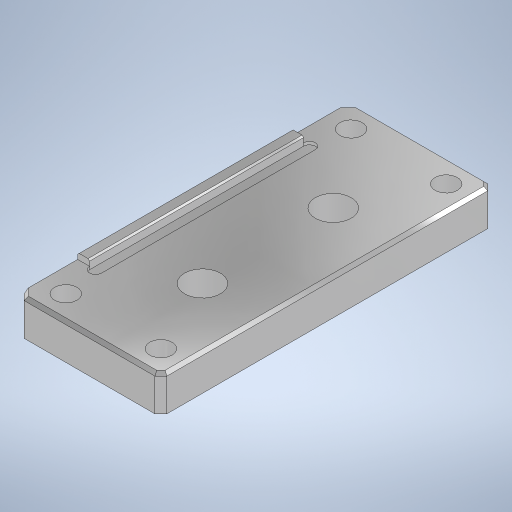
# Autodesk Inventor part: Base - Stationary
Saved by Autodesk Inventor 2023.2 (Build 272271000, 271)
## iProperties
Created: 2024-03-01
Part Number: Base - Stationary
Material: Aluminum 6061
Document SubType Name: Modeling
Designer: Nathan Cai
Density: 2.7 g/cm^3
Appearance: Aluminum - Flat
Author: Nathan Cai
Autodesk Inventor part; units mm, degrees
ref_plane "YZ Plane" through (0, 0, 0) normal (1, 0, 0) x (0, 1, 0)
ref_plane "XZ Plane" through (0, 0, 0) normal (0, 1, 0) x (-1, 0, 0)
ref_plane "XY Plane" through (0, 0, 0) normal (0, 0, 1) x (1, 0, 0)
sketch "Sketch1" plane through (0, 0, 0) normal (0, 1, 0) x (-1, 0, 0)
  line L0 (19.05, 44.45) -> (-19.05, 44.45)
  line L1 (-19.05, 44.45) -> (-19.05, -44.45)
  line L2 (-19.05, -44.45) -> (19.05, -44.45)
  line L3 (19.05, -44.45) -> (19.05, 44.45)
  line L4 (19.05, 44.45) -> (-19.05, -44.45) construction
  line L5 (-19.05, 44.45) -> (19.05, -44.45) construction
  line L6 (19.05, 0) -> (-19.05, 0) construction
  line L7 (0, 44.45) -> (0, -44.45) construction
  line L8 (19.05, 38.1) -> (-19.05, 38.1) construction
  circle A0 centre (-12.7, 38.1) radius 3
  circle A1 centre (12.7, 38.1) radius 3
  circle A2 centre (-12.7, -38.1) radius 3
  circle A3 centre (12.7, -38.1) radius 3
  line L9 (-19.05, -17.4625) -> (19.05, -17.4625) construction
  circle A4 centre (-3.175, -17.4625) radius 4.7942
  line L10 (-19.05, 17.4625) -> (19.05, 17.4625) construction
  circle A5 centre (-3.175, 17.4625) radius 4.7942
  point P0 (0, 0)
  dimension "d0" = 38.1
  dimension "d1" = 88.9
  dimension "d2" = 6.35
  dimension "d3" = 6
  dimension "d4" = 6.35
  dimension "d7" = 25.4
  dimension "d10" = 76.2
  dimension "d33" = 26.9875
  dimension "d34" = 9.5885
  dimension "d35" = 15.875
  constraints: 22 end point, 7 point on line, 6 centre point, 6 midpoint, 3 perpendicular, 3 symmetric about line, 2 horizontal, 2 parallel, 1 vertical, 7 other
  measures "d0" distance of L2.end L1.end
  measures "d1" distance between parallel lines of L2 L0
  measures "d2" distance between parallel lines of L0 L8
  measures "d3" diameter of A0
  measures "d4" distance from line of L1 A0.centre
  measures "d7" distance of A0.centre A1.centre
  measures "d10" distance of A0.centre A2.centre
  measures "d33" distance between parallel lines of L2 L9
  measures "d34" diameter of A4
  measures "d35" distance from line of L1 A4.centre
extrude "Extrusion1" add sketch "Sketch1" along normal blind 9.525
sketch "Sketch2" plane through (0, 9.525, 0) normal (0, 1, 0) x (1, 0, 0)
  line L0 (-19.05, 44.45) -> (-19.05, -44.45) projected
  line L1 (-19.05, 0) -> (19.05, 0) construction
  line L2 (19.05, -44.45) -> (19.05, 44.45) projected
  line L3 (-19.05, -28.575) -> (-15.875, -28.575)
  line L4 (-15.875, -28.575) -> (-15.875, 28.575)
  line L5 (-15.875, 28.575) -> (-19.05, 28.575)
  line L6 (-19.05, 28.575) -> (-19.05, -28.575)
  line L7 (-19.05, -28.575) -> (-15.875, 28.575) construction
  line L8 (-15.875, -28.575) -> (-19.05, 28.575) construction
  point P0 (0, 0)
  point P1 (-17.4625, 0)
  dimension "d15" = 3.175
  dimension "d16" = 57.15
  dimension "d36" = 0
  constraints: 14 end point, 4 midpoint, 2 parallel, 1 horizontal, 1 perpendicular, 1 point on line
  measures "d15" distance of L5.end L4.end
  measures "d16" distance of L4.end L3.end
  measures "d36" distance between parallel lines of L0 L6
extrude "Extrusion2" add sketch "Sketch2" along normal blind 1.5875
chamfer "Chamfer1" distance 1.5875 angle 45 4 edges at (-19.05, 4.7625, -44.45) (-19.05, 4.7625, 44.45) (19.05, 4.7625, 44.45) (19.05, 4.7625, -44.45)
chamfer "Chamfer2" distance 0.3969 angle 45 2 edges at (-19.05, 11.1125, 0) (-15.875, 11.1125, 0)
chamfer "Chamfer3" distance 0.7937 angle 45 7 edges at (0, 9.525, -44.45) (18.2562, 9.525, -43.6562) (-18.2563, 9.525, -43.6562) (-18.2562, 9.525, 43.6562) (0, 9.525, 44.45) (18.2562, 9.525, 43.6562) (19.05, 9.525, 0)
sketch "Sketch3" plane through (0, 9.525, 0) normal (0, 1, 0) x (1, 0, 0)
  line L0 (-19.05, 42.8625) -> (-19.05, -42.8625) projected
  line L1 (-19.05, 0) -> (19.05, 0) construction
  line L2 (19.05, -42.8625) -> (19.05, 42.8625) projected
  line L3 (-14.2875, -28.575) -> (-14.2875, 28.575) construction
  line L4 (-12.7, -28.575) -> (-12.7, 28.575)
  line L5 (-15.875, 28.575) -> (-15.875, -28.575)
  arc A0 (-15.875, -28.575) -> (-12.7, -28.575) centre (-14.2875, -28.575) ccw
  arc A1 (-12.7, 28.575) -> (-15.875, 28.575) centre (-14.2875, 28.575) ccw
  point P0 (0, 0)
  point P1 (-14.2875, 0)
  dimension "d30" = 3.175
  constraints: 11 end point, 4 point on circle, 4 tangent, 3 midpoint, 2 centre point, 1 parallel, 1 perpendicular, 1 point on line
  measures "d30" diameter of A1
extrude "Extrusion3" cut sketch "Sketch3" against normal blind 0.7937
body "Solid1"
